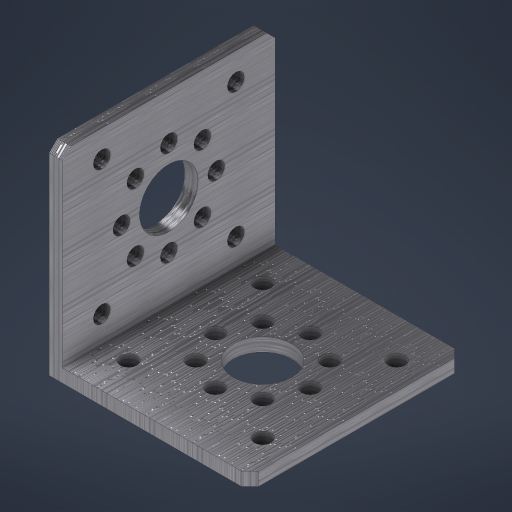
# Autodesk Inventor part: Arashtrix 48mm x 48mm L-Bracket
Saved by Autodesk Inventor 2024 (Build 280153000, 153)
## iProperties
Created: 2023-10-17
Part Number: Arashtrix 48mm x 48mm L-Bracket
Material: Generic
Document SubType Name: Modeling
Designer: avsar
Density: 1 g/cm^3
Appearance: Machined 03
Author: avsar
Autodesk Inventor part; units mm, degrees
ref_plane "YZ Plane" through (0, 0, 0) normal (1, 0, 0) x (0, 1, 0)
ref_plane "XZ Plane" through (0, 0, 0) normal (0, 1, 0) x (-1, 0, 0)
ref_plane "XY Plane" through (0, 0, 0) normal (0, 0, 1) x (1, 0, 0)
sketch "Sketch1" plane through (0, 0, 0) normal (0, 0, 1) x (1, 0, 0)
  line L0 (0, 48) -> (0, 0)
  line L1 (0, 0) -> (48, 0)
  line L2 (48, 0) -> (48, 3.175)
  line L3 (0, 48) -> (3.175, 48)
  line L4 (3.175, 48) -> (3.175, 3.175)
  line L5 (3.175, 3.175) -> (48, 3.175)
  dimension "d0" = 48
  dimension "d1" = 48
  dimension "d2" = 3.175
  dimension "d3" = 3.175
  constraints: 12 end point, 3 perpendicular, 2 horizontal, 1 coincident, 1 vertical
  measures "d0" distance of L0.start L0.end
  measures "d1" distance of L0.end L1.end
  measures "d2" distance of L1.end L2.end
  measures "d3" distance of L0.start L3.end
extrude "Extrusion1" add sketch "Sketch1" along normal mid plane 50.8
sketch "Sketch2" plane through (3.175, 3.175, 25.4) normal (0, 1, 0) x (1, 0, 0)
  line L0 (0, 50.8) -> (0, 0) construction
  line L1 (44.825, 0) -> (0, 0) construction
  line L2 (44.825, 50.8) -> (44.825, 0) construction
  line L3 (0, 50.8) -> (44.825, 50.8) construction
  line L4 (-3.175, 0) -> (44.825, 0) projected
  line L5 (22.4125, 0) -> (22.4125, 50.8) construction
  line L6 (0, 25.4) -> (44.825, 25.4) construction
  circle A0 centre (22.4125, 25.4) radius 7
  circle A1 centre (14.4125, 33.4) radius 2
  circle A2 centre (11.0988, 25.4) radius 2
  circle A3 centre (14.4125, 17.4) radius 2
  circle A4 centre (22.4125, 14.0863) radius 2
  circle A5 centre (30.4125, 17.4) radius 2
  circle A6 centre (33.7262, 25.4) radius 2
  circle A7 centre (30.4125, 33.4) radius 2
  circle A8 centre (22.4125, 36.7137) radius 2
  circle A9 centre (38.4125, 9.4) radius 2
  circle A10 centre (6.4125, 9.4) radius 2
  circle A11 centre (38.4125, 41.4) radius 2
  circle A12 centre (6.4125, 41.4) radius 2
  point P0 (-3.175, 25.4)
  dimension "d6" = 14
  dimension "d7" = 4
  dimension "d8" = 8
  dimension "d9" = 8
  dimension "d12" = 360
  dimension "d14" = 4
  dimension "d15" = 16
  dimension "d16" = 16
  constraints: 13 centre point, 6 midpoint, 4 end point, 3 symmetric about line, 1 coincident, 1 point on line, 20 other
  measures "d6" diameter of A0
  measures "d7" diameter of A1
  measures "d8" horizontal distance of A1.centre point (22.413, 25.4)
  measures "d9" horizontal distance of A1.centre point (22.413, 25.4)
  measures "d14" diameter of A9
  measures "d15" horizontal distance of point (22.413, 25.4) A9.centre
  measures "d16" horizontal distance of A0.centre A9.centre
extrude "Extrusion2" cut sketch "Sketch2" against normal through all
sketch "Sketch3" plane through (3.175, 3.175, 25.4) normal (1, 0, 0) x (0, 0, -1)
  line L0 (50.8, 44.825) -> (0, 44.825) construction
  line L1 (0, 0) -> (0, 44.825) construction
  line L2 (50.8, 0) -> (0, 0) construction
  line L3 (50.8, 44.825) -> (50.8, 0) construction
  line L4 (50.8, 44.825) -> (0, 44.825) projected
  line L5 (25.4, 44.825) -> (25.4, 0) construction
  line L6 (0, 22.4125) -> (50.8, 22.4125) construction
  circle A0 centre (25.4, 22.4125) radius 7
  circle A1 centre (33.4, 30.4125) radius 2
  circle A2 centre (25.4, 33.7262) radius 2
  circle A3 centre (17.4, 30.4125) radius 2
  circle A4 centre (14.0863, 22.4125) radius 2
  circle A5 centre (17.4, 14.4125) radius 2
  circle A6 centre (25.4, 11.0988) radius 2
  circle A7 centre (33.4, 14.4125) radius 2
  circle A8 centre (36.7137, 22.4125) radius 2
  circle A9 centre (9.4, 38.4125) radius 2
  circle A10 centre (9.4, 6.4125) radius 2
  circle A11 centre (41.4, 38.4125) radius 2
  circle A12 centre (41.4, 6.4125) radius 2
  point P0 (25.4, -3.175)
  dimension "d19" = 14
  dimension "d20" = 4
  dimension "d21" = 8
  dimension "d22" = 8
  dimension "d25" = 360
  dimension "d27" = 4
  dimension "d28" = 16
  dimension "d29" = 16
  constraints: 13 centre point, 6 midpoint, 4 end point, 3 symmetric about line, 20 other
  measures "d19" diameter of A0
  measures "d20" diameter of A1
  measures "d21" horizontal distance of point (25.4, 22.413) A1.centre
  measures "d22" horizontal distance of A0.centre A1.centre
  measures "d27" diameter of A9
  measures "d28" horizontal distance of A9.centre point (25.4, 22.413)
  measures "d29" horizontal distance of point (25.4, 22.413) A9.centre
extrude "Extrusion3" cut sketch "Sketch3" against normal through all
chamfer "Chamfer1" distance 2 angle 45 4 edges at (1.5875, 48, 25.4) (1.5875, 48, -25.4) (48, 1.5875, 25.4) (48, 1.5875, -25.4)
body "Solid1"
